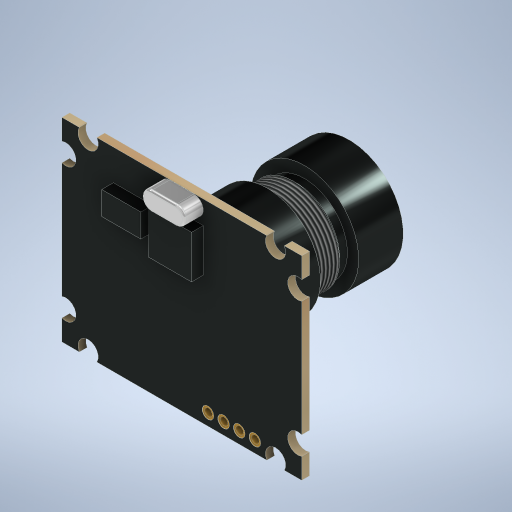
# Autodesk Inventor part: CAMERA
Saved by Autodesk Inventor 2023 (Build 270158000, 158)
## iProperties
Created: 2023-03-15
Part Number: CAMERA
Material: Generic
Document SubType Name: Modeling
Designer: Amos Yu
Density: 1 g/cm^3
Appearance: Gunmetal - Polished
Author: Amos Yu
Autodesk Inventor part; units mm, degrees
ref_plane "YZ Plane" through (0, 0, 0) normal (1, 0, 0) x (0, 1, 0)
ref_plane "XZ Plane" through (0, 0, 0) normal (0, 1, 0) x (-1, 0, 0)
sketch "Sketch1" plane through (0, 0, 0) normal (0, 0, 1) x (1, 0, 0)
  arc A0 (-15.35, 7.4) -> (-15.35, 9.8) centre (-14.85, 8.6) ccw
  arc A1 (-13.1258, 12.45) -> (-10.8742, 12.45) centre (-12, 11.8) ccw
  line L0 (0, -12.45) -> (0, 12.45) construction
  line L1 (-15.35, 0) -> (15.35, 0) construction
  arc A2 (15.35, 9.8) -> (15.35, 7.4) centre (14.85, 8.6) ccw
  arc A3 (10.8742, 12.45) -> (13.1258, 12.45) centre (12, 11.8) ccw
  arc A4 (-15.35, -9.8) -> (-15.35, -7.4) centre (-14.85, -8.6) ccw
  arc A5 (-10.8742, -12.45) -> (-13.1258, -12.45) centre (-12, -11.8) ccw
  arc A6 (13.1258, -12.45) -> (10.8742, -12.45) centre (12, -11.8) ccw
  arc A7 (15.35, -7.4) -> (15.35, -9.8) centre (14.85, -8.6) ccw
  line L2 (-15.35, 9.8) -> (-15.35, 12.45)
  line L3 (-15.35, 12.45) -> (-13.1258, 12.45)
  line L4 (-10.8742, 12.45) -> (10.8742, 12.45)
  line L5 (13.1258, 12.45) -> (15.35, 12.45)
  line L6 (15.35, 12.45) -> (15.35, 9.8)
  line L7 (15.35, 7.4) -> (15.35, -7.4)
  line L8 (15.35, -9.8) -> (15.35, -12.45)
  line L9 (15.35, -12.45) -> (13.1258, -12.45)
  line L10 (10.8742, -12.45) -> (-10.8742, -12.45)
  line L11 (-13.1258, -12.45) -> (-15.35, -12.45)
  line L12 (-15.35, -12.45) -> (-15.35, -9.8)
  line L13 (-15.35, -7.4) -> (-15.35, 7.4)
  point P0 (0, 0)
  dimension "d0" = 30.7
  dimension "d1" = 24.9
  dimension "d2" = 2.6
  dimension "d3" = 14.85
  dimension "d4" = 8.6
  dimension "d5" = 2.6
  dimension "d6" = 11.8
  dimension "d7" = 12
  dimension "d8" = 14.8
  dimension "d9" = 2.65
  dimension "d10" = 2.2242
  dimension "d11" = 21.7483
  dimension "d12" = 2.2242
  dimension "d13" = 2.65
  dimension "d14" = 14.8
  dimension "d15" = 2.65
  dimension "d16" = 21.7483
  dimension "d17" = 2.2242
  dimension "d18" = 2.65
  constraints: 28 end point, 18 parallel, 16 point on circle, 12 perpendicular, 8 centre point, 6 symmetric about line, 4 midpoint, 3 horizontal, 1 horizontal alignment, 1 vertical alignment, 6 other
  measures "d0" distance of L8.end L11.end
  measures "d1" distance of L5.end L8.end
  measures "d2" diameter of A0
  measures "d3" horizontal distance of point (0, 0) A0.centre
  measures "d4" vertical distance of point (0, 0) A0.centre
  measures "d5" diameter of A1
  measures "d6" vertical distance of point (0, 0) A1.centre
  measures "d7" horizontal distance of point (0, 0) A1.centre
  measures "d8" distance of L13.start L13.end
  measures "d9" distance of L11.end L12.end
  measures "d10" distance of L11.start L11.end
  measures "d11" distance of L10.start L10.end
  measures "d12" distance of L8.end L9.end
  measures "d13" distance of L8.start L8.end
  measures "d14" distance of L7.start L7.end
  measures "d15" distance of L5.end L6.end
  measures "d16" distance of L4.start L4.end
  measures "d17" distance of L2.end L3.end
  measures "d18" distance of L2.start L2.end
extrude "Extrusion1" add sketch "Sketch1" along normal blind 1
sketch "Sketch2" plane through (0, 0, 1) normal (0, 0, 1) x (1, 0, 0)
  line L0 (-8.75, 8.5) -> (-3.75, 8.5)
  line L1 (-3.75, 8.5) -> (-3.75, 5.5)
  line L2 (-3.75, 5.5) -> (-8.75, 5.5)
  line L3 (-8.75, 5.5) -> (-8.75, 8.5)
  line L4 (-2.75, 9.5) -> (2.75, 9.5)
  line L5 (2.75, 9.5) -> (2.75, 4)
  line L6 (2.75, 4) -> (-2.75, 4)
  line L7 (-2.75, 4) -> (-2.75, 9.5)
  line L8 (-1.55, 11.2) -> (1.55, 11.2) construction
  line L9 (-1.55, 10) -> (1.55, 10)
  line L10 (1.55, 12.4) -> (-1.55, 12.4)
  arc A0 (-1.55, 12.4) -> (-1.55, 10) centre (-1.55, 11.2) ccw
  arc A1 (1.55, 10) -> (1.55, 12.4) centre (1.55, 11.2) ccw
  line L11 (10.8742, 12.45) -> (-10.8742, 12.45) projected
  point P0 (0, 0)
  point P1 (0, 4)
  point P2 (0, 11.2)
  point P3 (0, 12.4)
  point P4 (2.75, 11.2)
  point P5 (2.75, 6.75)
  point P6 (0, 12.45)
  dimension "d21" = 5.5
  dimension "d22" = 5.5
  dimension "d23" = 4
  dimension "d24" = 0
  dimension "d25" = 1
  dimension "d26" = 5
  dimension "d27" = 3
  dimension "d28" = 1
  dimension "d29" = 1.2
  dimension "d36" = 0.05
  constraints: 24 end point, 5 midpoint, 5 parallel, 5 point on circle, 4 tangent, 3 horizontal, 2 centre point, 2 perpendicular, 2 vertical alignment
  measures "d21" distance of L4.end L5.end
  measures "d22" distance of L4.start L4.end
  measures "d23" distance from line of point (0, 0) L6
  measures "d24" horizontal distance of point (0, 4) point (0, 0)
  measures "d25" distance between parallel lines of L7 L1
  measures "d26" distance of L0.start L0.end
  measures "d27" distance of L2.end L0.start
  measures "d28" distance between parallel lines of L4 L0
  measures "d29" distance between parallel lines of L10 L8
  measures "d36" distance between parallel lines of L11 L10
extrude "Extrusion2" add sketch "Sketch2" along normal blind 1.5 contours L0 L1 L2 L3 | L4 L5 L6 L7
extrude "Extrusion3" add sketch "Sketch2" along normal blind 2.4 contours A0 L10 A1 L9
fillet "Fillet1" radius 0.3 4 edges at (-2.75, 11.2, 3.4) (0, 10, 3.4) (2.75, 11.2, 3.4) (0, 12.4, 3.4)
sketch "Sketch3" plane through (0, 0, 0) normal (0, 0, -1) x (-1, 0, 0)
  point P0 (0, 0)
sketch "Sketch4" plane through (0, 0, 0) normal (0, 0, -1) x (-1, 0, 0)
  line L0 (-6.4, 6.4) -> (6.4, 6.4)
  line L1 (6.4, -6.4) -> (-6.4, -6.4)
  line L2 (-6.4, 6.4) -> (6.4, -6.4) construction
  line L3 (6.4, 6.4) -> (-6.4, -6.4) construction
  arc A0 (-8.9, 1.85) -> (-8.9, -1.85) centre (-8.9, 0) ccw
  line L4 (-8.9, 1.85) -> (-6.4, 1.85)
  line L5 (-8.9, -1.85) -> (-6.4, -1.85)
  line L6 (-6.4, -6.4) -> (-6.4, -1.85)
  line L7 (-6.4, 1.85) -> (-6.4, 6.4)
  line L8 (0, 6.4) -> (0, -6.4) construction
  arc A1 (8.9, -1.85) -> (8.9, 1.85) centre (8.9, 0) ccw
  line L9 (8.9, 1.85) -> (6.4, 1.85)
  line L10 (8.9, -1.85) -> (6.4, -1.85)
  line L11 (6.4, 6.4) -> (6.4, 1.85)
  line L12 (6.4, -1.85) -> (6.4, -6.4)
  circle A2 centre (-8.9, 0) radius 0.75
  circle A3 centre (8.9, 0) radius 0.75
  point P0 (0, 0)
  dimension "d37" = 12.8
  dimension "d38" = 12.8
  dimension "d39" = 3.7
  dimension "d40" = 8.9
  dimension "d41" = 1.5
  dimension "d42" = 1.5
  constraints: 26 end point, 5 parallel, 5 symmetric about line, 4 centre point, 4 midpoint, 4 point on circle, 3 horizontal, 2 coincident, 2 perpendicular, 2 tangent, 1 horizontal alignment, 1 other
  measures "d37" distance of L1.start L1.end
  measures "d38" distance of L0.end L1.start
  measures "d39" diameter of A0
  measures "d40" distance of point (0, 0) A0.centre
  measures "d41" diameter of A2
  measures "d42" diameter of A3
extrude "Extrusion4" add sketch "Sketch4" along normal blind 2.5
sketch "Sketch5" plane through (0, 0, 0) normal (0, 1, 0) x (-1, 0, 0)
  line L0 (0, 0) -> (0, -19.5)
  line L1 (0, 0) -> (6.85, 0)
  line L2 (6.85, 0) -> (6.85, -9.9)
  line L3 (6.85, -9.9) -> (5.9, -9.9)
  line L4 (5.9, -9.9) -> (5.9, -13.3)
  line L5 (5.9, -13.3) -> (5.5, -13.7)
  line L6 (5.5, -13.7) -> (5.5, -14.7)
  line L7 (5.5, -14.7) -> (6.95, -14.7)
  line L8 (6.95, -14.7) -> (6.95, -20.4)
  line L9 (6.95, -20.4) -> (5.35, -20.4)
  arc A0 (5.35, -20.4) -> (0, -19.5) centre (0, -35.8514) ccw
  dimension "d45" = 13.7
  dimension "d46" = 11.8
  dimension "d47" = 11
  dimension "d48" = 13.9
  dimension "d49" = 1.6
  dimension "d50" = 9.9
  dimension "d51" = 5.7
  dimension "d52" = 20.4
  dimension "d53" = 1
  dimension "d54" = 135
  dimension "d56" = 19.5
  constraints: 20 end point, 5 perpendicular, 2 horizontal, 2 point on circle, 1 centre point, 1 coincident, 1 line through centre, 1 parallel, 1 vertical
  measures "d45" diameter of L2 L0
  measures "d46" diameter of L4 L0
  measures "d47" diameter of L6 L0
  measures "d48" diameter of L8 L0
  measures "d49" distance of L8.end L9.end
  measures "d50" distance of L1.end L2.end
  measures "d51" distance of L7.end L8.end
  measures "d52" vertical distance of L8.end L1.end
  measures "d53" distance of L5.end L6.end
  measures "d54" angle of L6 L5
  measures "d56" distance of L0.start L0.end
revolve "Revolution1" add sketch "Sketch5" angle 360 about axis through (0, 0, 0) along (0, 0, -1)
thread "Thread1" size "M12x0.5" class "6g" standard "ANSI Metric M Profile" full length
sketch "Sketch6" plane through (0, 0, 1) normal (0, 0, 1) x (1, 0, 0)
  circle A0 centre (9.35, -10.95) radius 0.5
  circle A1 centre (9.35, -10.95) radius 0.75
  line L0 (-10.8742, -12.45) -> (10.8742, -12.45) projected
  line L1 (15.35, -12.45) -> (15.35, -9.8) projected
  circle A2 centre (7.35, -10.95) radius 0.5
  circle A3 centre (7.35, -10.95) radius 0.75
  circle A4 centre (5.35, -10.95) radius 0.5
  circle A5 centre (5.35, -10.95) radius 0.75
  circle A6 centre (3.35, -10.95) radius 0.5
  circle A7 centre (3.35, -10.95) radius 0.75
  point P0 (0, 0)
  dimension "d60" = 1
  dimension "d61" = 1.5
  dimension "d62" = 1.5
  dimension "d63" = 6
  dimension "d66" = 2
  constraints: 8 centre point, 4 coincident, 1 horizontal, 12 other
  measures "d60" diameter of A0
  measures "d61" diameter of A1
  measures "d62" distance from line of L0 A0.centre
  measures "d63" distance from line of L1 A0.centre
  measures "d66" distance of A0.centre A2.centre
extrude "Extrusion5" cut sketch "Sketch6" against normal through all contours A0 | A2 | A4 | A6
extrude "Extrusion6" cut sketch "Sketch6" against normal blind 0.05
ref_plane "Work Plane1" through (0, 0, 0.5) normal (0, 0, -1) x (-1, 0, 0)
mirror "Mirror1" about plane through (0, 0, 0.5) normal (0, 0, -1) of "Extrusion6"
extrude "Extrusion7" add sketch "Sketch4" along normal blind 2 contours A2 | A3
body "Solid1"
